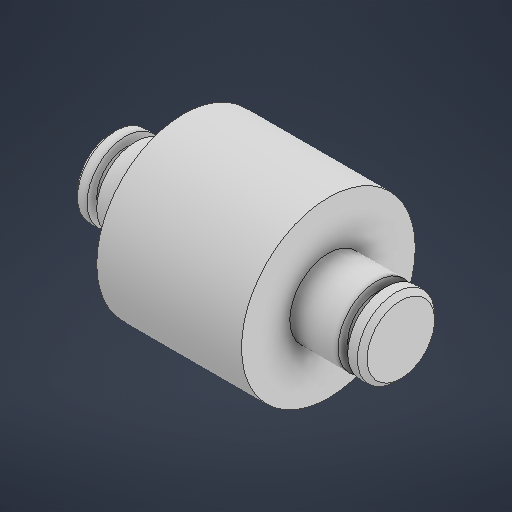
# Autodesk Inventor part: Hinge
Saved by Autodesk Inventor 2025.4 (Build 294407000, 407)
## iProperties
Created: 2026-05-27
Part Number: Hinge
Material: Generic
Document SubType Name: Modeling
Designer: VuQuan
Density: 1 g/cm^3
Appearance: Default
Author: VuQuan
Autodesk Inventor part; units mm, degrees
ref_plane "YZ Plane" through (0, 0, 0) normal (1, 0, 0) x (0, 1, 0)
ref_plane "XZ Plane" through (0, 0, 0) normal (0, 1, 0) x (-1, 0, 0)
ref_plane "XY Plane" through (0, 0, 0) normal (0, 0, 1) x (1, 0, 0)
sketch "Sketch1" plane through (0, 0, 0) normal (0, 0, 1) x (1, 0, 0)
  line L0 (0, 0) -> (15, 0)
  line L1 (15, 0) -> (15, 3.5)
  line L2 (14.5, 4) -> (13.5, 4)
  line L3 (13.5, 4) -> (13.5, 3)
  line L4 (13.5, 3) -> (12.5, 3)
  line L5 (12.5, 3) -> (12.5, 4)
  line L6 (12.5, 4) -> (7.5, 4)
  line L7 (7.5, 4) -> (7.5, 9)
  line L8 (7.5, 9) -> (0, 9)
  line L9 (0, 9) -> (0, 0) construction
  line L10 (15, 3.5) -> (14.5, 4)
  line L11 (-15, 0) -> (-15, 3.5)
  line L12 (-14.5, 4) -> (-13.5, 4)
  line L13 (-13.5, 4) -> (-13.5, 3)
  line L14 (-13.5, 3) -> (-12.5, 3)
  line L15 (-12.5, 3) -> (-12.5, 4)
  line L16 (-12.5, 4) -> (-7.5, 4)
  line L17 (-7.5, 4) -> (-7.5, 9)
  line L18 (-7.5, 9) -> (0, 9)
  line L19 (-15, 3.5) -> (-14.5, 4)
  line L20 (0, 0) -> (-15, 0)
  point P0 (15, 4)
  point P1 (-15, 4)
  dimension "d0" = 8
  dimension "d1" = 6
  dimension "d2" = 1
  dimension "d3" = 7.5
  dimension "d4" = 30
  dimension "d5" = 18
  dimension "d6" = 0.5
  dimension "d7" = 0.5
  constraints: 42 end point, 10 symmetric about line, 7 perpendicular, 4 point on line, 2 horizontal, 1 collinear, 1 parallel
  measures "d0" diameter of L6 L0
  measures "d1" diameter of L4 L0
  measures "d2" distance between parallel lines of L3 L5
  measures "d3" distance between parallel lines of L1 L7
  measures "d4" diameter of L1 L9
  measures "d5" diameter of L8 L0
  measures "d6" distance of L1.end point (15, 4)
  measures "d7" distance of L2.start point (15, 4)
revolve "Revolution1" add sketch "Sketch1" angle 360 about axis through (0, 0, 0) along (-1, 0, 0)
equation "\"d7\" = d6"
body "Solid1"
